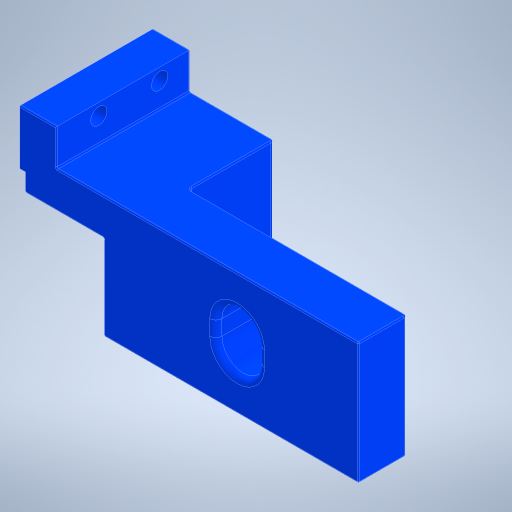
# Autodesk Inventor part: mount_right
Saved by Autodesk Inventor 2023.4 (Build 274418000, 418)
## iProperties
Created: 2022-05-25
Part Number: mount_right
Material: Generic
Document SubType Name: Modeling
Designer: SB13FLLT004
Density: 1 g/cm^3
Appearance: Default(1)
Author: SB13FLLT004
Autodesk Inventor part; units mm, degrees
ref_plane "YZ Plane" through (0, 0, 0) normal (1, 0, 0) x (0, 1, 0)
ref_plane "XZ Plane" through (0, 0, 0) normal (0, 1, 0) x (-1, 0, 0)
ref_plane "XY Plane" through (0, 0, 0) normal (0, 0, 1) x (1, 0, 0)
derived "main_manifold_8v_v02.ipt"
sketch "Sketch:MM: main inlet" plane through (0, 0, 0) normal (1, 0, 0) x (0, 1, 0)
  line L0 (20.32, 0) -> (0, 0)
  line L1 (0, 0) -> (0, -27.94)
  line L2 (0, -27.94) -> (20.32, -27.94)
  line L3 (20.32, -27.94) -> (20.32, 0)
  point P0 (13.97, -15.24)
sketch "Sketch:MM: mounting screws:1" plane through (0, 0, 0) normal (-1, 0, 0) x (0, 0, 1)
  line L0 (-27.94, 0) -> (-27.94, 16.256)
  line L1 (-21.59, 5.08) -> (-8.89, 5.08) construction
  point P0 (0, 0)
  point P1 (-15.24, 13.97)
  point P2 (-15.24, 5.08)
sketch "Sketch: reference" plane through (0, 0, 0) normal (0, 0, 1) x (1, 0, 0)
  line L0 (-24.765, -0.4572) -> (-2.159, -0.4572)
  line L1 (-2.159, -0.4572) -> (-2.159, -4.2672)
  line L2 (-2.159, -4.2672) -> (-24.765, -4.2672)
  line L3 (-24.765, -4.2672) -> (-24.765, -0.4572)
  line L4 (-24.765, 20.32) -> (0, 20.32)
  line L5 (0, 0) -> (-24.765, 0)
  line L6 (-24.765, 0) -> (-24.765, 20.32)
  line L7 (0, 20.32) -> (0, 0) projected
  line L8 (-10.6362, -4.2672) -> (-10.6362, -8.8392)
  line L9 (-10.6362, -8.8392) -> (-1.016, -8.8392)
  line L10 (-1.016, -8.8392) -> (-1.016, -25.2984)
  dimension "d43" = 3.81
  dimension "d45" = 0.4572
  dimension "d47" = 22.606
  dimension "d48" = 2.159
  dimension "d49" = 4.572
  dimension "d50" = 1.016
  dimension "d51" = 8.4772
  constraints: 20 end point, 9 perpendicular, 1 coincident, 1 collinear, 1 point on line
  measures "d43" distance of L0.end L1.end
  measures "d45" distance between parallel lines of L0 L5
  measures "d47" distance of L1.end L2.end
  measures "d48" distance between parallel lines of L7 L1
  measures "d49" distance of L8.start L8.end
  measures "d50" distance between parallel lines of L10 L7
  measures "d51" distance between parallel lines of L8 L1
sketch "Sketch: side profile" plane through (0, 0, 0) normal (0, 0, 1) x (1, 0, 0)
  line L0 (-1.712, -7.62) -> (38.288, -7.62) construction
  line L1 (38.288, -7.62) -> (38.288, -47.62) construction
  line L2 (38.288, -47.62) -> (-1.712, -47.62) construction
  line L3 (-1.712, -47.62) -> (-1.712, -7.62) construction
  line L4 (11.43, -12.065) -> (1.016, -12.065)
  line L5 (1.016, -12.065) -> (1.016, 0)
  line L6 (1.016, 0) -> (25.146, 0)
  line L7 (70.734, 0) -> (70.734, -25.4)
  line L8 (25.146, -25.4) -> (25.146, -7.62)
  line L9 (25.146, -7.62) -> (11.43, -7.62)
  line L10 (11.43, -7.62) -> (11.43, -12.065)
  line L11 (11.43, -8.89) -> (-1.712, -8.89) construction
  line L12 (25.146, -8.89) -> (38.288, -8.89) construction
  line L13 (0, -3.81) -> (0, 0)
  line L14 (0, 0) -> (1.016, 0)
  line L15 (1.016, -7.62) -> (11.43, -7.62)
  line L16 (70.734, -25.4) -> (25.146, -25.4)
  line L17 (0, -3.81) -> (1.016, -3.81)
  line L18 (0, 20.32) -> (0, 0) construction
  line L19 (-2.159, -4.2672) -> (-24.765, -4.2672) construction
  line L20 (-24.765, -0.4572) -> (-2.159, -0.4572) construction
  line L21 (-2.159, -0.4572) -> (-2.159, -4.2672) construction
  line L22 (-24.765, 20.32) -> (0, 20.32) construction
  line L23 (0, 0) -> (-24.765, 0) construction
  line L24 (-1.016, -8.8392) -> (-1.016, -25.2984) construction
  line L25 (-10.6362, -8.8392) -> (-1.016, -8.8392) construction
  line L26 (-10.6362, -4.2672) -> (-10.6362, -8.8392) construction
  line L27 (25.4, 22.4728) -> (25.4, 6.8361) construction
  line L28 (25.146, 0) -> (25.146, -7.62)
  line L29 (25.4, 10.8949) -> (65.4, 10.8949) construction
  line L30 (65.4, 10.8949) -> (65.4, -32.4037) construction
  line L31 (65.4, -32.4037) -> (25.4, -32.4037) construction
  line L32 (25.4, -32.4037) -> (25.4, 10.8949) construction
  arc A0 (49.845, -11.1125) -> (40.955, -11.1125) centre (45.4, -11.1125) ccw
  arc A1 (40.955, -14.2875) -> (49.845, -14.2875) centre (45.4, -14.2875) ccw
  line L33 (40.955, -11.1125) -> (40.955, -14.2875)
  line L34 (49.845, -11.1125) -> (49.845, -14.2875)
  line L35 (65.654, 0) -> (65.654, -25.4)
  line L36 (70.734, 0) -> (25.146, 0)
  line L37 (25.146, 0) -> (25.146, 0)
  line L38 (17.526, 0) -> (17.526, -25.4)
  line L39 (17.526, -25.4) -> (25.146, -25.4)
  point P0 (1.016, -5.08)
  point P1 (0, 0)
  point P2 (0, -3.8003)
  point P3 (38.288, -27.62)
  point P4 (45.4, 10.8949)
  point P5 (49.845, -12.7)
  point P6 (70.734, -12.7)
  point P7 (17.526, -7.62)
  dimension "d1" = 40
  dimension "d2" = 13.142
  dimension "d3" = 7.62
  dimension "d22" = 1.016
  dimension "d25" = 4.445
  dimension "d30" = 1.27
  dimension "d34" = -1.712
  dimension "d52" = 3.81
  dimension "space_bt_olfa_and_post" = 25.4
  dimension "d56" = 12.065
  dimension "d64" = 10.414
  dimension "d65" = 11.43
  dimension "d68" = 17.78
  dimension "d70" = 40
  dimension "d73" = 3.175
  dimension "d74" = 4.445
  dimension "d78" = 5.08
  dimension "d79" = 0.254
  dimension "d82" = 25.146
  dimension "d83" = 0.254
  dimension "d84" = 25.4
  dimension "d86" = 7.62
  constraints: 62 end point, 19 perpendicular, 10 point on line, 5 collinear, 5 horizontal, 4 midpoint, 4 point on circle, 4 tangent, 2 centre point, 2 equal length, 2 parallel, 1 horizontal alignment, 1 vertical, 1 vertical alignment
  measures "d1" distance of L0.start L0.end
  measures "d2" distance of L12.start L12.end
  measures "d3" distance between parallel lines of L6 L9
  measures "d22" distance between parallel lines of L13 L5
  measures "d25" distance of L9.end L4.start
  measures "d30" distance between parallel lines of L0 L12
  measures "d34" distance between parallel lines of L13 L3
  measures "d52" distance of L13.start L13.end
  measures "space_bt_olfa_and_post" distance between parallel lines of L27 L18
  measures "d56" distance between parallel lines of L4 L6
  measures "d64" distance of L4.start L4.end
  measures "d65" distance between parallel lines of L10 L13
  measures "d68" distance between parallel lines of L16 L0
  measures "d70" distance of L29.start L29.end
  measures "d73" distance of L34.start L34.end
  measures "d74" radius of A0
  measures "d78" distance between parallel lines of L7 L35
  measures "d79" distance between parallel lines of L35 L30
  measures "d82" distance between parallel lines of L28 L13
  measures "d83" distance between parallel lines of L32 L28
  measures "d84" distance of L7.start L7.end
  measures "d86" distance of L38.end L8.start
sketch "Sketch: MM holes" plane through (0, 0, 0) normal (1, 0, 0) x (0, 1, 0)
  line L0 (20.32, -27.94) -> (20.32, 0) construction
  line L1 (20.32, 0) -> (0, 0) construction
  line L2 (0, -27.94) -> (20.32, -27.94) construction
  line L3 (0, 0) -> (0, -27.94) construction
  circle A0 centre (5.08, -8.89) radius 1.2065 construction
  line L4 (7.5565, 0) -> (0, 0)
  line L5 (0, 0) -> (0, -27.94)
  line L6 (0, -27.94) -> (7.5565, -27.94)
  line L7 (7.5565, -27.94) -> (7.5565, 0)
  circle A1 centre (13.97, -15.24) radius 4.3688 construction
  line L8 (20.32, -15.24) -> (17.145, -20.7393) construction
  line L9 (17.145, -20.7393) -> (10.795, -20.7393) construction
  line L10 (10.795, -20.7393) -> (7.62, -15.24) construction
  line L11 (7.62, -15.24) -> (10.795, -9.7407) construction
  line L12 (10.795, -9.7407) -> (17.145, -9.7407) construction
  line L13 (17.145, -9.7407) -> (20.32, -15.24) construction
  line L14 (20.32, -15.24) -> (7.62, -15.24) construction
  line L15 (7.5565, 0) -> (12.0015, 0)
  line L16 (12.0015, 0) -> (12.0015, -2.54)
  line L17 (10.0965, -4.445) -> (7.5565, -4.445)
  line L18 (7.5565, -27.94) -> (12.0015, -27.94)
  line L19 (12.0015, -27.94) -> (12.0015, -25.4)
  line L20 (10.0965, -23.495) -> (7.5565, -23.495)
  arc A2 (12.0015, -25.4) -> (10.0965, -23.495) centre (10.0965, -25.4) ccw
  arc A3 (10.0965, -4.445) -> (12.0015, -2.54) centre (10.0965, -2.54) ccw
  line L21 (12.0015, -2.54) -> (7.5565, -4.1876)
  line L22 (12.0015, -25.4) -> (7.5565, -22.0114)
  point P0 (5.08, -21.59)
  point P1 (13.97, -15.24)
  dimension "d5" = 2.413
  dimension "d21" = 7.5565
  dimension "d89" = 8.7376
  dimension "d94" = 120
  dimension "d95" = 120
  dimension "d96" = 6.35
  dimension "d98" = 4.445
  dimension "d99" = 1.905
  dimension "d102" = 2.54
  dimension "d105" = 4.445
  dimension "d106" = 4.445
  dimension "d107" = 2.54
  dimension "d108" = 0.0635
  constraints: 38 end point, 5 collinear, 5 equal length, 4 centre point, 4 point on circle, 4 point on line, 4 tangent, 3 coincident, 3 perpendicular, 2 horizontal, 2 parallel, 2 vertical, 2 vertical alignment, 1 equal radius, 1 midpoint
  measures "d5" diameter of A0
  measures "d21" distance of L5.end L6.end
  measures "d89" diameter of A1
  measures "d94" angle of L9 L8
  measures "d95" angle of L8 L13
  measures "d96" distance of L8.start L8.end
  measures "d98" distance from line of L2 L20.start
  measures "d99" radius of A2
  measures "d102" distance of L18.end L19.end
  measures "d105" distance from line of L1 L17.start
  measures "d106" distance between parallel lines of L7 L19
  measures "d107" distance from line of L1 L16.end
  measures "d108" distance from line of L7 L10.end
extrude "Ex: MM screws" add sketch "Sketch: MM holes" along normal blind 7.62 contours L7 L6 L5 L4
hole "Hole: MM screws (4-40)" at (0, 5.08, -8.89) at (0, 5.08, -21.59) direction (1, 0, 0) diameter 3.429 end through all
extrude "Ex: side profile" add sketch "Sketch: side profile" against normal up to surface (27.94 mm away) from surface at 0 contours L15 L5 L6 L38 L9 | L17 L13 L14 L5
extrude "Ex: inside face of item post" add sketch "Sketch: side profile" against normal up to surface (27.94 mm away) contours L38 L6 L28 L9 | L9 L8 L39 L38
extrude "Ex: front face of item post" add sketch "Sketch: side profile" against normal blind 10.16 contours L28 L36 L35 L16 L8 | L35 L36 L7 L16 | L34 A1 L33 A0
extrude "Ex: screw hole" cut sketch "Sketch: side profile" against normal through all contours L34 A1 L33 A0
fillet "Fillet1" radius 0.635 3 edges at (25.146, -12.7, -27.94) (25.146, -12.7, -10.16) (70.734, -12.7, -10.16)
fillet "Fillet2" radius 0.254 31 edges at (70.734, -12.7, 0) (44.13, -25.4, 0) (25.332, -25.4, -10.346) (25.146, -25.4, -19.05) (24.96, -25.4, -27.754) (21.0185, -25.4, -27.94) (70.548, -25.4, -9.974) (70.734, -25.4, -4.7625) (47.94, -25.4, -10.16) (70.548, 0, -9.974) (70.734, 0, -4.7625) (25.332, 0, -10.346) (25.146, 0, -19.05) (24.96, 0, -27.754) (16.0655, 0, -27.94) (47.94, 0, -10.16) (39.177, 0, 0) (17.526, -16.51, 0) (17.526, -25.4, -13.97) (17.526, -16.51, -27.94) (9.271, -7.62, -27.94) (7.62, 0, -13.97) (7.62, 3.7782, 0) (7.62, 3.7783, -27.94) (9.271, -7.62, 0) (1.016, -5.715, -27.94) (1.016, -5.715, 0) (3.81, 7.5565, 0) (3.81, 7.5565, -27.94) (17.526, -7.62, -13.97) (1.016, -7.62, -13.97)
fillet "Fillet3" radius 1.27 8 edges at (49.845, -12.7, -10.16) (45.4, -6.6675, -10.16) (40.955, -12.7, -10.16) (45.4, -18.7325, -10.16) (40.955, -12.7, 0) (45.4, -6.6675, 0) (49.845, -12.7, 0) (45.4, -18.7325, 0)
body "Solid1"
